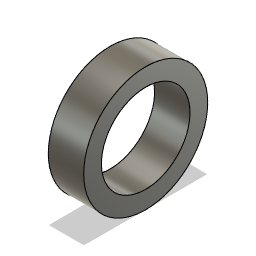
Spacer (Autodesk Fusion 360 design; units mm, degrees)
Autodesk Fusion 360 part; units mm, degrees
sketch "Sketch1" plane through (0, 0, 0) normal (0, 0, 1) x (1, 0, 0)
  line L0 (-10, 0) -> (10, 0)
  line L1 (-5, 12.5) -> (5, 12.5)
  line L2 (-5, 17.5) -> (5, 17.5)
  line L3 (-5, 12.5) -> (-5, 17.5)
  line L4 (5, 12.5) -> (5, 17.5)
  line L5 (-5, 12.5) -> (5, 12.5)
  line L6 (-5, 17.5) -> (5, 17.5)
revolve "Revolve1" add sketch "Sketch1" angle 360 about axis through (-10, 0, 0) along (1, 0, 0)
equation "angle = 360.0 deg"
